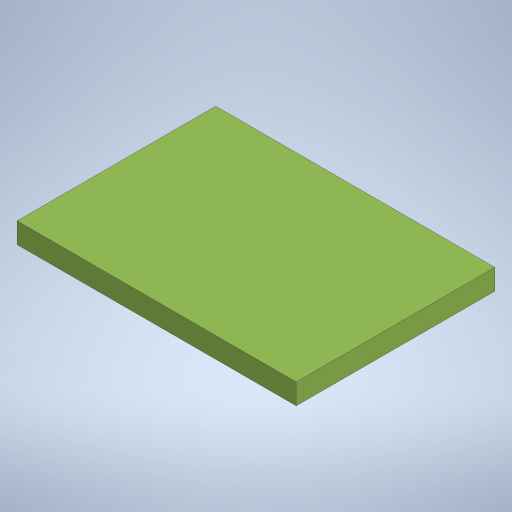
# Autodesk Inventor part: sensor
Saved by Autodesk Inventor 2023 (Build 270158000, 158)
## iProperties
Created: 2023-10-14
Part Number: sensor
Material: Generic
Document SubType Name: Modeling
Designer: Gage
Density: 1 g/cm^3
Appearance: Default
Author: Gage
Autodesk Inventor part; units mm, degrees
ref_plane "YZ Plane" through (0, 0, 0) normal (1, 0, 0) x (0, 1, 0)
ref_plane "XZ Plane" through (0, 0, 0) normal (0, 1, 0) x (-1, 0, 0)
ref_plane "XY Plane" through (0, 0, 0) normal (0, 0, 1) x (1, 0, 0)
sketch "Sketch1" plane through (0, 0, 0) normal (0, 1, 0) x (-1, 0, 0)
  line L0 (11.3347, -8.0645) -> (-11.3347, -8.0645)
  line L1 (-11.3347, -8.0645) -> (-11.3347, 8.0645)
  line L2 (-11.3347, 8.0645) -> (11.3347, 8.0645)
  line L3 (11.3347, 8.0645) -> (11.3347, -8.0645)
  point P0 (0, 0)
  point P1 (0, -8.0645)
  point P2 (-11.3348, 0)
  dimension "d2" = 22.6695
  dimension "d3" = 16.129
  constraints: 8 end point, 2 midpoint, 2 parallel, 1 horizontal, 1 horizontal alignment, 1 perpendicular, 1 vertical alignment
  measures "d2" distance of L1.end L2.end
  measures "d3" distance of L0.end L1.end
extrude "Extrusion1" add sketch "Sketch1" along normal blind 1.6764
body "Solid1"
